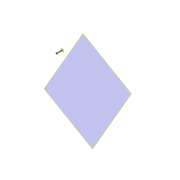
# Autodesk Inventor part: BOLT
Saved by Autodesk Inventor 2016 (Build 200138000, 138)
## iProperties
Created: 2016-03-31
Part Number: BOLT
Material: Stainless Steel
Document SubType Name: Modeling
Designer: admin
Density: 8.08 g/cm^3
Appearance: Semi-Polished
Author: admin
Autodesk Inventor part; units mm, degrees
ref_plane "YZ Plane" through (0, 0, 0) normal (1, 0, 0) x (0, 1, 0)
ref_plane "XZ Plane" through (0, 0, 0) normal (0, 1, 0) x (-1, 0, 0)
ref_plane "XY Plane" through (0, 0, 0) normal (0, 0, 1) x (1, 0, 0)
ref_plane "Work Plane1" through (-112.0932, 314.7709, -230.7555) normal (0, 1, 0) x (-0.5, 0, -0.866)
sketch "Sketch1" plane through (-112.0932, 314.7709, -230.7555) normal (0, 1, 0) x (-0.5, 0, -0.866)
  circle A0 centre (-2, 232) radius 4
  point P0 (-255.8867, 18.3022)
  dimension "d0" = 8
  constraints: 1 centre point
  measures "d0" diameter of A0
extrude "Extrusion1" add sketch "Sketch1" along normal blind 36.5
sketch "Sketch2" plane through (-312.0111, 314.7709, -113.0235) normal (0, -1, 0) x (1, 0, 0)
  circle A0 centre (0, 0) radius 4 projected
  arc A1 (5.5, 3.4641) -> (5.5, -3.4641) centre (0, 0) ccw
  line L0 (5.5, -3.4641) -> (5.5, 3.4641)
  point P0 (312.0111, 113.0235)
  dimension "d3" = 13
  dimension "d29" = 5.5
  constraints: 2 end point, 2 point on circle, 1 centre point, 1 coincident, 1 vertical
  measures "d3" diameter of A1
  measures "d29" distance from line of A0.centre L0
extrude "Extrusion2" add sketch "Sketch2" along normal blind 4.5 contours A0 | L0 A1
thread "Thread1" size "M8x1.25" class "6g" standard "ANSI Metric M Profile" length 21
ref_plane "Work Plane2" through (-312.0111, 351.2709, -113.0235) normal (0, 1, 0) x (1, 0, 0)
sketch "Sketch4" plane through (-312.0111, 351.2709, -113.0235) normal (0, 1, 0) x (1, 0, 0)
  circle A0 centre (0, 0) radius 3.7 projected
  line L0 (-11, 1) -> (10, 1)
  line L1 (-11, -1) -> (13, -1)
  line L2 (-11, 1) -> (3, 13)
  line L3 (3, 13) -> (10, 1)
  line L4 (-11, -1) -> (8, -15)
  line L5 (8, -15) -> (13, -1)
  point P0 (312.0111, -113.0235)
  dimension "d16" = 1
  dimension "d17" = 1
  constraints: 12 end point
  measures "d16" distance from line of A0.centre L0
  measures "d17" distance from line of A0.centre L1
extrude "Extrusion4" cut sketch "Sketch4" against normal blind 0.9 contours L0 A0 | A0 L0 L2 L3 | L1 L5 L4 A0 | A0 L1
sketch "Sketch5" plane through (-112.0932, 351.2709, -230.7555) normal (0, 1, 0) x (0.866, 0, -0.5)
  arc A0 (-229.415, -4.6472) -> (-228.415, -2.9151) centre (-232, -2) ccw projected
  point P0 (-18.3022, -255.8867)
hole "Hole1" at (-312.0111, 351.2709, -113.0235) direction (0, -1, 0) diameter 2.459 depth 10.8 tip angle 118 countersink diameter 5 countersink angle 90 thread size "M3x0.5" class "6H" standard "ISO Metric profile"
sketch "Sketch6" plane through (-112.0932, 351.2709, -230.7555) normal (0, 1, 0) x (0.866, 0, -0.5)
  arc A0 (-229.415, -4.6472) -> (-228.415, -2.9151) centre (-232, -2) ccw projected
  circle A1 centre (-232, -2) radius 10.2956
  point P0 (-18.3022, -255.8867)
  constraints: 1 centre point, 1 coincident
extrude "Extrusion5" cut sketch "Sketch6" against normal blind 0.2
sketch "Sketch7" plane through (-112.0932, 351.0709, -230.7555) normal (0, 1, 0) x (0.866, 0, -0.5)
  arc A0 (-230.7063, -3.9016) -> (-229.7063, -2.1696) centre (-232, -2) ccw projected
  circle A1 centre (-232, -2) radius 3.4
  circle A2 centre (-232, -2) radius 1.2295 projected
  circle A3 centre (-232, -2) radius 5.5146
  point P0 (-18.3022, -255.8867)
  dimension "d30" = 6.8
  constraints: 2 centre point, 2 coincident
  measures "d30" diameter of A1
extrude "Extrusion6" cut sketch "Sketch7" against normal blind 1 contours A3
chamfer "Chamfer2" distance 0.3 angle 45 1 edges at (-310.0111, 350.0709, -109.5594)
body "Solid1"
